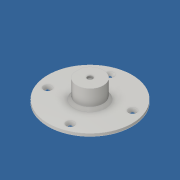
# Autodesk Inventor part: OberArmMagnet
Saved by Autodesk Inventor 2016 (Build 200138000, 138)
## iProperties
Created: 2015-09-18
Part Number: OberArmMagnet
Material: ABS-Kunststoff
Document SubType Name: Modeling
Designer: 4ndreas
Density: 1.06 g/cm^3
Appearance: Glatt - weiß
Mass: 29.4816 g
Surface Area: 182.587 cm^2
Volume: 27.8128 cm^3
Author: 4ndreas
Autodesk Inventor part; units mm, degrees
ref_plane "YZ Plane" through (0, 0, 0) normal (1, 0, 0) x (0, 1, 0)
ref_plane "XZ Plane" through (0, 0, 0) normal (0, 1, 0) x (-1, 0, 0)
ref_plane "XY Plane" through (0, 0, 0) normal (0, 0, 1) x (1, 0, 0)
sketch "Skizze1" plane through (0, 0, 0) normal (0, 0, 1) x (1, 0, 0)
  circle A0 centre (-35.2385, -12.8258) radius 2.1 projected
  circle A1 centre (-12.8258, 35.2385) radius 2.1 projected
  circle A2 centre (12.8258, -35.2385) radius 2.1 projected
  circle A3 centre (35.2385, 12.8258) radius 2.1 projected
  circle A4 centre (0, 0) radius 25 projected
  circle A5 centre (0, 0) radius 45 projected
  circle A6 centre (0, 0) radius 47.5 projected
  circle A7 centre (0, 0) radius 8.4675
  point P0 (0, 0)
  constraints: 1 centre point, 1 coincident
extrude "Extrusion1" add sketch "Skizze1" along normal blind 3 contours A4 | A5 | A6 | A7
sketch "Skizze2" plane through (0, 0, 3) normal (0, 0, 1) x (1, 0, 0)
  circle A0 centre (0, 0) radius 15
  dimension "d2" = 30
  constraints: 1 centre point, 1 coincident
  measures "d2" diameter of A0
extrude "Extrusion2" add sketch "Skizze2" along normal blind 21
sketch "Skizze3" plane through (0, 0, 24) normal (0, 0, 1) x (1, 0, 0)
  circle A0 centre (0, 0) radius 3
  dimension "d7" = 6
  constraints: 1 centre point, 1 coincident
  measures "d7" diameter of A0
extrude "Extrusion3" cut sketch "Skizze3" against normal blind 2.5
sketch "Skizze4" plane through (0, 0, 0) normal (0, 0, -1) x (-1, 0, 0)
  circle A0 centre (0, 0) radius 15 projected
  circle A1 centre (0, 0) radius 11
  dimension "d8" = 4
  constraints: 1 centre point, 1 coincident
  measures "d8" radial gap between concentric circles of A0 A1
extrude "Extrusion4" cut sketch "Skizze4" against normal blind 20 contours A1
sketch "Skizze5" plane through (0, 0, 0) normal (0, 0, -1) x (-1, 0, 0)
  circle A0 centre (0, 0) radius 11 projected
  circle A1 centre (-35.2385, 12.8258) radius 2.1 projected
  circle A2 centre (-12.8258, -35.2385) radius 2.1 projected
  circle A3 centre (12.8258, 35.2385) radius 2.1 projected
  circle A4 centre (35.2385, -12.8258) radius 2.1 projected
  circle A5 centre (0, 0) radius 47.5 projected
  line L0 (10, -4.5826) -> (10, 4.5826)
  dimension "d11" = 10
  constraints: 2 end point, 2 point on circle, 1 vertical
  measures "d11" distance from line of L0 point (0, 0)
extrude "Extrusion5" add sketch "Skizze5" against normal up to surface (20 mm away) contours A0 L0 picked at (10.1839, -1.0361)
sketch "Skizze6" plane through (-10, -4.5826, 0) normal (1, 0, 0) x (0, 0, -1)
  line L0 (-20, 0) -> (-20, 9.1652) projected
  line L1 (0, 0) -> (-20, 0) projected
  line L2 (0, 9.1652) -> (0, 0) projected
  line L3 (-20, 9.1652) -> (0, 9.1652) projected
  line L4 (-3, -10.4174) -> (-3, 19.5826) projected
  line L5 (-3, 15.3083) -> (-3, 19.5083) projected
  line L6 (-3, -32.7559) -> (-3, -28.5559) projected
  line L7 (-3, 37.721) -> (-3, 41.921) projected
  line L8 (-3, -10.3432) -> (-3, -6.1432) projected
  line L9 (-3, 52.0826) -> (-3, -42.9174) projected
  line L10 (-3, 0) -> (-20, 0)
  line L11 (-20, 0) -> (-20, 9.1652)
  line L12 (-20, 9.1652) -> (-3, 9.1652)
  line L13 (-3, 9.1652) -> (-3, 0)
  point P0 (0, 4.5826)
  constraints: 8 end point, 3 point on line, 2 parallel, 1 collinear, 1 horizontal, 1 perpendicular
extrude "Extrusion6" cut sketch "Skizze6" against normal blind 20 contours L0 L3 L4 L1
sketch "Skizze7" plane through (0, 0, 20) normal (0, 0, -1) x (-1, 0, 0)
  arc A0 (10, 4.5826) -> (10, -4.5826) centre (0, 0) ccw projected
  line L0 (10, -4.5826) -> (14.2829, -4.5826) projected
  arc A1 (14.2829, -4.5826) -> (14.2829, 4.5826) centre (0, 0) ccw projected
  line L1 (10, 4.5826) -> (14.2829, 4.5826) projected
  line L2 (14.2829, 4.5826) -> (14.2829, -4.5826)
  constraints: 2 end point, 1 vertical
extrude "Extrusion7" cut sketch "Skizze7" against normal blind 20 contours A1 L2
chamfer "Fase1" distance 3 angle 45 1 edges at (15, 0, 3)
chamfer "Fase2" distance 2.5 angle 45 4 edges at (-14.9258, 35.2385, 3) (33.1385, 12.8258, 3) (10.7258, -35.2385, 3) (-37.3385, -12.8258, 3)
